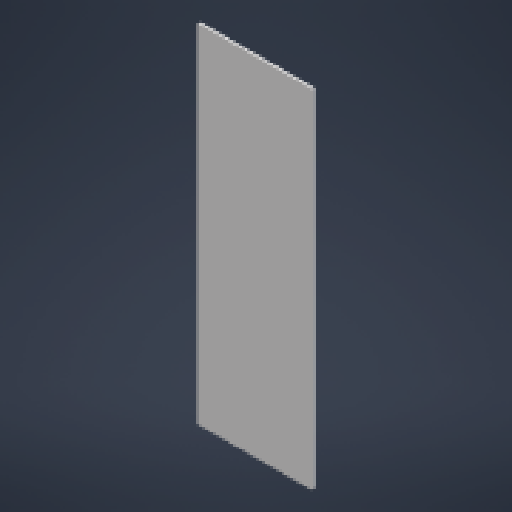
# Autodesk Inventor part: zpanel
Saved by Autodesk Inventor 2025.1 (Build 291241020, 241B)
## iProperties
Created: 2024-09-23
Part Number: zpanel
Material: Generic
Document SubType Name: Modeling
Designer: techn
Density: 1 g/cm^3
Appearance: Default
Author: techn
Autodesk Inventor part; units mm, degrees
ref_plane "YZ Plane" through (0, 0, 0) normal (1, 0, 0) x (0, 1, 0)
ref_plane "XZ Plane" through (0, 0, 0) normal (0, 1, 0) x (-1, 0, 0)
ref_plane "XY Plane" through (0, 0, 0) normal (0, 0, 1) x (1, 0, 0)
sketch "Sketch1" plane through (0, 0, 0) normal (0, 0, 1) x (1, 0, 0)
  line L0 (0, -445) -> (-144, -445) projected
  arc A0 (-147, -442) -> (-144, -445) centre (-144, -442) ccw projected
  line L1 (-147, -442) -> (-147, 2) projected
  arc A1 (-144, 5) -> (-147, 2) centre (-144, 2) ccw projected
  line L2 (-144, 5) -> (0, 5) projected
  arc A2 (3, 2) -> (0, 5) centre (0, 2) ccw projected
  line L3 (3, 2) -> (3, -442) projected
  arc A3 (0, -445) -> (3, -442) centre (0, -442) ccw projected
  point P0 (0, 0)
extrude "Extrusion1" add sketch "Sketch1" along normal blind 3
body "Solid1"
